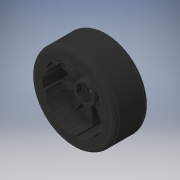
# Autodesk Inventor part: Roue
Saved by Autodesk Inventor 2019 (Build 230136000, 136)
## iProperties
Created: 2019-07-30
Part Number: Roue
Material: Caoutchouc
Document SubType Name: Modeling
Designer: Sébastien DI MERCURIO
Density: 0.93 g/cm^3
Appearance: Caoutchouc - Noir
Author: Sébastien DI MERCURIO
Autodesk Inventor part; units mm, degrees
ref_plane "YZ Plane" through (0, 0, 0) normal (1, 0, 0) x (0, 1, 0)
ref_plane "XZ Plane" through (0, 0, 0) normal (0, 1, 0) x (-1, 0, 0)
ref_plane "XY Plane" through (0, 0, 0) normal (0, 0, 1) x (1, 0, 0)
sketch "Esquisse1" plane through (0, 0, 0) normal (0, 0, 1) x (1, 0, 0)
  circle A0 centre (0, 0) radius 32.5
  dimension "d0" = 65
  constraints: 1 centre point, 1 coincident
  measures "d0" diameter of A0
extrude "Extrusion1" add sketch "Esquisse1" along normal blind 26
sketch "Esquisse3" plane through (0, 0, 26) normal (0, 0, 1) x (1, 0, 0)
  circle A0 centre (0, 0) radius 22.5
  dimension "d6" = 45
  constraints: 1 centre point, 1 coincident
  measures "d6" diameter of A0
extrude "Extrusion3" cut sketch "Esquisse3" against normal blind 12.5
sketch "Esquisse4" plane through (0, 0, 13.5) normal (0, 0, 1) x (1, 0, 0)
  circle A0 centre (0, 0) radius 8
  dimension "d9" = 16
  constraints: 1 centre point, 1 coincident
  measures "d9" diameter of A0
extrude "Extrusion4" add sketch "Esquisse4" along normal blind 4
sketch "Esquisse2" plane through (0, 0, 26) normal (0, 0, 1) x (1, 0, 0)
  circle A0 centre (0, 0) radius 2
  dimension "d3" = 4
  constraints: 1 centre point, 1 coincident
  measures "d3" diameter of A0
extrude "Extrusion2" cut sketch "Esquisse2" against normal through all
sketch "Esquisse5" plane through (0, 0, 17.5) normal (0, 0, 1) x (1, 0, 0)
  line L0 (0, 6.9282) -> (6, 3.4641)
  line L1 (6, 3.4641) -> (6, -3.4641)
  line L2 (6, -3.4641) -> (0, -6.9282)
  line L3 (0, -6.9282) -> (-6, -3.4641)
  line L4 (-6, -3.4641) -> (-6, 3.4641)
  line L5 (-6, 3.4641) -> (0, 6.9282)
  point P0 (0, 0)
  point P1 (0, 0)
  dimension "d12" = 12
  constraints: 12 end point, 1 coincident, 1 vertical alignment, 13 other
  measures "d12" distance from line of L3 L0.start
extrude "Extrusion5" cut sketch "Esquisse5" against normal blind 4
sketch "Esquisse6" plane through (0, 0, 0) normal (0, 0, -1) x (-1, 0, 0)
  circle A0 centre (0, 0) radius 11.25
  dimension "d15" = 22.5
  constraints: 1 centre point, 1 coincident
  measures "d15" diameter of A0
extrude "Extrusion6" cut sketch "Esquisse6" against normal blind 10
chamfer "Chanfrein1" distance 10 angle 45 1 edges at (11.25, 0, 0)
sketch "Esquisse7" plane through (0, 0, 10) normal (0, 0, -1) x (-1, 0, 0)
  circle A0 centre (0, 0) radius 5
  dimension "d21" = 10
  constraints: 1 centre point, 1 coincident
  measures "d21" diameter of A0
extrude "Extrusion7" cut sketch "Esquisse7" against normal blind 2
sketch "Esquisse8" plane through (0, 0, 0) normal (0, 0, -1) x (-1, 0, 0)
  line L0 (23.4733, 5) -> (8.3688, 1.5)
  line L1 (8.3688, -1.5) -> (23.4733, -5)
  arc A0 (23.4733, -5) -> (23.4733, 5) centre (0.009, 0) ccw
  arc A1 (8.3688, -1.5) -> (8.3688, 1.5) centre (0.009, 0) ccw
  point P0 (0, 0)
  dimension "d26" = 3
  dimension "d27" = 1.5
  dimension "d28" = 10
  dimension "d29" = 5
  constraints: 4 end point, 4 point on circle, 2 centre point, 1 coincident
  measures "d26" distance of L0.end L1.start
  measures "d27" vertical distance of L0.end point (0, 0)
  measures "d28" distance of L1.end L0.start
  measures "d29" vertical distance of point (0, 0) L0.start
extrude "Extrusion8" cut sketch "Esquisse8" against normal through all
pattern_circular "Réseau circulaire1" count 10 over 360 about axis through (0, 0, 26) along (0, 0, -1) of "Extrusion8"
fillet "Congé1" radius 3 2 edges at (-32.5, 0, 0) (-32.5, 0, 26)
equation "\"d27\" = 0.5 * d26"
equation "\"d29\" = 0.5 * d28"
